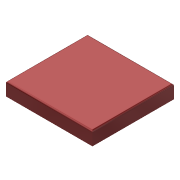
# Autodesk Inventor part: RomeoSudoController
Saved by Autodesk Inventor 2018 (Build 220112000, 112)
## iProperties
Created: 2018-10-17
Part Number: RomeoSudoController
Material: Generic
Document SubType Name: Modeling
Designer: Vulnic
Density: 1 g/cm^3
Appearance: Default
Author: Vulnic
Autodesk Inventor part; units mm, degrees
ref_plane "YZ Plane" through (0, 0, 0) normal (1, 0, 0) x (0, 1, 0)
ref_plane "XZ Plane" through (0, 0, 0) normal (0, 1, 0) x (-1, 0, 0)
ref_plane "XY Plane" through (0, 0, 0) normal (0, 0, 1) x (1, 0, 0)
sketch "Sketch1" plane through (0, 0, 0) normal (0, 1, 0) x (-1, 0, 0)
  line L0 (0, 0) -> (-89, 0)
  line L1 (-89, 0) -> (-89, 84)
  line L2 (-89, 84) -> (0, 84)
  line L3 (0, 84) -> (0, 0)
  dimension "d0" = 89
  dimension "d1" = 84
  constraints: 8 end point, 2 parallel, 1 horizontal, 1 perpendicular
  measures "d0" distance of L0.start L0.end
  measures "d1" distance of L2.end L0.start
extrude "Extrusion1" add sketch "Sketch1" along normal blind 14
fillet "Fillet1" radius 2 4 edges at (44.5, 14, 0) (0, 14, 42) (89, 14, 42) (44.5, 14, 84)
sketch "Sketch2" plane through (0, 14, 0) normal (0, 1, 0) x (1, 0, 0)
  line L0 (89, 0) -> (0, 0) projected
  line L1 (6.9319, 0) -> (15.3203, 0)
  line L2 (15.3203, 0) -> (15.3203, -11.7863)
  line L3 (15.3203, -11.7863) -> (6.9319, -11.7863)
  line L4 (6.9319, -11.7863) -> (6.9319, 0)
  line L5 (20.9884, 0) -> (29.3768, 0)
  line L6 (29.3768, 0) -> (29.3768, -11.7863)
  line L7 (29.3768, -11.7863) -> (20.9884, -11.7863)
  line L8 (20.9884, -11.7863) -> (20.9884, 0)
  line L9 (67.6628, 0) -> (76.0512, 0)
  line L10 (76.0512, 0) -> (76.0512, -11.7863)
  line L11 (76.0512, -11.7863) -> (67.6628, -11.7863)
  line L12 (67.6628, -11.7863) -> (67.6628, 0)
  line L13 (7, -84.0181) -> (15.3884, -84.0181)
  line L14 (15.3884, -84.0181) -> (15.3884, -72.2317)
  line L15 (15.3884, -72.2317) -> (7, -72.2317)
  line L16 (7, -72.2317) -> (7, -84.0181)
  line L17 (89, -84) -> (0, -84) projected
  constraints: 32 end point, 7 parallel, 6 equal length, 4 horizontal, 4 perpendicular, 3 point on line
extrude "Extrusion2" cut sketch "Sketch2" against normal blind 5
body "Solid1"
